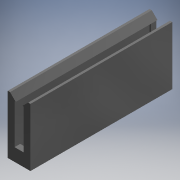
# Autodesk Inventor part: cord holder
Saved by Autodesk Inventor 2019 (Build 230136000, 136)
## iProperties
Part Number: cord holder
Material: Generic
Document SubType Name: Modeling
Designer: Delta
Appearance: Default
Author: Delta
Autodesk Inventor part; units mm, degrees
ref_plane "YZ Plane" through (0, 0, 0) normal (1, 0, 0) x (0, 1, 0)
sketch "Sketch1" plane through (0, 0, 0) normal (0, 1, 0) x (-1, 0, 0)
  line L0 (0, 0) -> (5.08, 0)
  line L1 (5.08, 0) -> (5.08, -31.75)
  line L2 (5.08, -31.75) -> (0, -31.75)
  line L3 (0, -31.75) -> (0, 0)
  dimension "d0" = 5.08
  dimension "d1" = 31.75
  constraints: 8 end point, 3 perpendicular, 1 horizontal
  measures "d0" distance of L0.start L0.end
  measures "d1" distance of L0.end L1.end
extrude "Extrusion1" add sketch "Sketch1" along normal blind 1.5875
sketch "Sketch6" plane through (0, 1.5875, 0) normal (0, 1, 0) x (1, 0, 0)
  line L0 (-5.08, 0) -> (0, 0) projected
  line L1 (0, 31.75) -> (-5.08, 31.75) projected
  line L2 (0, 0) -> (-1.27, 0)
  line L3 (-1.27, 0) -> (-1.27, 31.75)
  line L4 (-1.27, 31.75) -> (0, 31.75)
  line L5 (0, 31.75) -> (0, 0)
  line L6 (-5.08, 31.75) -> (-5.08, 0) projected
  line L7 (-5.08, 0) -> (-3.81, 0)
  line L8 (-3.81, 0) -> (-3.81, 31.75)
  line L9 (-3.81, 31.75) -> (-5.08, 31.75)
  line L10 (-5.08, 31.75) -> (-5.08, 0)
  dimension "d19" = 31.75
  dimension "d20" = 1.27
  dimension "d21" = 31.75
  dimension "d22" = 1.27
  constraints: 16 end point, 4 parallel, 2 horizontal, 2 perpendicular, 1 point on line
  measures "d19" distance between parallel lines of L0 L1
  measures "d20" distance of L3.end L4.end
  measures "d21" distance between parallel lines of L0 L4
  measures "d22" distance between parallel lines of L6 L8
extrude "Extrusion7" add sketch "Sketch6" along normal blind 11.43 contours L6 L1 L8 L0 | L3 L1 L5 L0
sketch "Sketch7" plane through (0, 1.5875, 0) normal (0, 1, 0) x (1, 0, 0)
  line L0 (-3.81, 0) -> (-1.27, 0) projected
  line L1 (-3.81, 31.75) -> (-3.81, 0) projected
  line L2 (-1.27, 0) -> (-3.81, 0)
  line L3 (-3.81, 0) -> (-3.81, 1.27)
  line L4 (-3.81, 1.27) -> (-1.27, 1.27)
  line L5 (-1.27, 1.27) -> (-1.27, 0)
  point P0 (0, 0)
  dimension "d25" = 1.27
  constraints: 8 end point, 2 parallel, 1 horizontal, 1 perpendicular, 1 point on line
  measures "d25" distance of L2.end L3.end
extrude "Extrusion8" add sketch "Sketch7" along normal blind 1.27
sketch "Sketch8" plane through (-1.27, 1.5875, -31.75) normal (-1, 0, 0) x (0, 0, 1)
  line L0 (0, 11.43) -> (31.75, 11.43) projected
  line L1 (0, 11.43) -> (31.75, 11.43)
  line L2 (31.75, 11.43) -> (31.75, 10.16)
  line L3 (31.75, 10.16) -> (0, 10.16)
  line L4 (0, 10.16) -> (0, 11.43)
  point P0 (31.75, -1.5875)
  dimension "d28" = 31.75
  dimension "d29" = 1.27
  constraints: 8 end point, 2 parallel, 1 horizontal, 1 perpendicular
  measures "d28" distance of L2.end L3.end
  measures "d29" distance of L1.end L2.end
extrude "Extrusion9" add sketch "Sketch8" along normal blind 0.508
chamfer "Chamfer1" distance 1.27 angle 45 1 edges at (-1.778, 13.0175, -15.875)
sketch "Sketch9" plane through (-1.27, 1.5875, -31.75) normal (-1, 0, 0) x (0, 0, 1)
  line L0 (30.48, 1.27) -> (31.75, 1.27) projected
  line L1 (31.75, 1.27) -> (30.48, 1.27)
  line L2 (30.48, 1.27) -> (30.48, 10.16)
  line L3 (30.48, 10.16) -> (31.75, 10.16)
  line L4 (31.75, 10.16) -> (31.75, 1.27)
  point P0 (31.75, -1.5875)
  dimension "d35" = 1.27
  dimension "d36" = 8.89
  constraints: 8 end point, 2 parallel, 1 horizontal, 1 perpendicular
  measures "d35" distance of L2.end L3.end
  measures "d36" distance of L1.end L2.end
extrude "Extrusion10" add sketch "Sketch9" along normal blind 0.254
ref_plane "Work Plane5" through (-5.08, 0, -15.875) normal (0, 0, 1) x (1, 0, 0)
ref_plane "Work Plane6" through (-2.54, 0, -31.75) normal (-1, 0, 0) x (0, 0, 1)
mirror "Mirror4" about plane through (-2.54, 0, -31.75) normal (-1, 0, 0) of "Extrusion9", "Chamfer1", "Extrusion10"
mirror "Mirror5" about plane through (-5.08, 0, -15.875) normal (0, 0, 1) of "Extrusion10", "Extrusion8"
sketch "Sketch10" plane through (-3.81, 1.5875, -1.27) normal (1, 0, 0) x (0, 0, -1)
  line L0 (30.48, 1.27) -> (29.21, 1.27)
  line L1 (29.21, 1.27) -> (29.21, 10.16)
  line L2 (29.21, 10.16) -> (30.48, 10.16)
  line L3 (30.48, 10.16) -> (30.48, 1.27)
  point P0 (-1.27, -1.5875)
  dimension "d39" = 1.27
  dimension "d40" = 8.89
  constraints: 8 end point, 2 parallel, 1 horizontal, 1 perpendicular
  measures "d39" distance of L1.end L2.end
  measures "d40" distance between parallel lines of L0 L2
extrude "Extrusion11" add sketch "Sketch10" along normal blind 0.254
equation "\"d21\" = d19"
equation "\"d22\" = d20"
body "Solid1"
